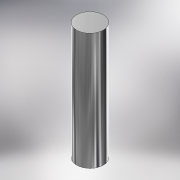
# Autodesk Inventor part: PistonRod
Saved by Autodesk Inventor 2013 SP2 (Build 170200200, 200)
## iProperties
Created: 2013-09-01
Part Number: PistonRod
Material: Steel
Document SubType Name: Modeling
Designer: Arto
Density: 7.85 g/cm^3
Author: Arto
Autodesk Inventor part; units mm, degrees
ref_plane "YZ Plane" through (0, 0, 0) normal (1, 0, 0) x (0, 1, 0)
ref_plane "XZ Plane" through (0, 0, 0) normal (0, 1, 0) x (-1, 0, 0)
ref_plane "XY Plane" through (0, 0, 0) normal (0, 0, 1) x (1, 0, 0)
sketch "Sketch1" plane through (0, 0, 0) normal (0, 0, 1) x (1, 0, 0)
  circle A0 centre (0, 0) radius 10 projected
extrude "Extrusion1" add sketch "Sketch1" against normal blind 110
sketch "Sketch2" plane through (0, 0, 0) normal (0, 0, 1) x (1, 0, 0)
  circle A0 centre (0, 0) radius 15
  dimension "d2" = 30
  constraints: 1 centre point, 1 coincident
  measures "d2" diameter of A0
extrude "Extrusion2" add sketch "Sketch2" against normal blind 5
chamfer "Chamfer1" distance 5 distance2 3 1 edges at (-15, 0, -5) measured on face at (-14.5, 0, -5)
body "Solid1"
